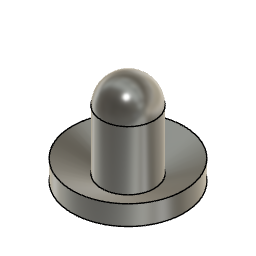
Pusher (Autodesk Fusion 360 design; units mm, degrees)
Autodesk Fusion 360 part; units mm, degrees
sketch "Sketch1" plane through (0, 0, 0) normal (0, 1, 0) x (1, 0, 0) in component "Pusher"
  line L0 (0, 0) -> (42.5, 0)
  line L1 (42.5, 0) -> (42.5, -15)
  line L2 (42.5, -15) -> (20, -5)
  line L3 (20, -5) -> (20, -50)
  arc A0 (0, -70) -> (20, -50) centre (0, -50) ccw
  line L4 (0, -70) -> (0, 0)
  dimension "d1" = 42.5
  dimension "d2" = 15
  dimension "d3" = 5
  dimension "d4" = 20
  dimension "d5" = 50
  dimension "d6" = 20
  constraint coincident L0.start L4.end
  constraint horizontal L0
  constraint perpendicular L0 L1
  constraint vertical L3
  constraint tangent L3 A0
  constraint vertical L0.start A0.start
  measures "d1" distance of L0.start L0.end
  measures "d2" distance of L0.end L1.end
  measures "d3" distance of L0 L2.end
  measures "d4" horizontal distance of L0.start L2.end
  measures "d5" distance of L0 L3.end
  measures "d6" vertical distance of L3.end A0.start
revolve "Revolve1" add sketch "Sketch1" angle 360 about axis through (0, 0, 70) along (0, 0, -1) in component "Pusher"
component "Pusher" placed x (1, 0, 0) y (0, 1, 0) z (0, 0, 1) at (0, 0, 0)
equation "d1 = ( 85 / 2 ) * 1 mm"
equation "d6 = d4"
